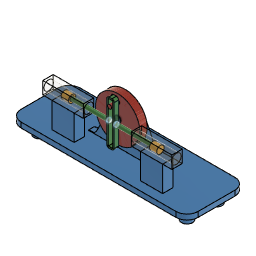
Scotch Yoke Mechanism (Autodesk Fusion 360 design; units mm, degrees)
Autodesk Fusion 360 part; units mm, degrees
note: some values were not read from the file. Set by a fixed rule: which face or edge a step refers to.
sketch "legs" plane through (0, 0, 0) normal (0, 0, 1) x (1, 0, 0) in component "Holder"
  circle A0 centre (-100, -20) radius 7.5
  circle A1 centre (100, -20) radius 7.5
  circle A2 centre (-100, 20) radius 7.5
  circle A3 centre (100, 20) radius 7.5
  dimension "d3" = 15
  dimension "d4" = 15
  dimension "d5" = 15
  dimension "d6" = 15
  measures "d3" diameter of A0
  measures "d4" diameter of A1
  measures "d5" diameter of A2
  measures "d6" diameter of A3
extrude "Extrude1" add sketch "legs" along normal blind 15 makes body 1 at (107.4627, 19.2532, 10) makes body 2 at (-92.5373, 19.2532, 10) makes body 3 at (107.4627, -20.7468, 10) makes body 4 at (-92.5373, -20.7468, 10) in component "Holder"
sketch "plank" plane through (0, 0, 15) normal (0, 0, 1) x (-1, 0, 0) in component "Holder"
  line L0 (120, 40) -> (-120, 40)
  line L1 (-120, 40) -> (-120, -40)
  line L2 (-120, -40) -> (120, -40)
  line L3 (120, -40) -> (120, 40)
  constraint horizontal L0
  constraint vertical L1
  constraint horizontal L2
  constraint vertical L3
extrude "Extrude2" add sketch "plank" along normal blind 7 bodies 1 2 3 4 in component "Holder"
fillet "Fillet1" radius 15 4 edges at (-120, -40, 18.5) (-120, 40, 18.5) (120, 40, 18.5) (120, -40, 18.5) on bodies 1 in component "Holder"
sketch "crank base" plane through (0, 0, 0) normal (0, 1, 0) x (1, 0, 0) in component "Holder"
  spline S0 degree 5 poles (-50, -22) (-49.5881, -22.201) (-48.7779, -22.5509) (-47.6039, -22.9192) (-46.1206, -23.0999) (-44.378, -22.949) (-42.6597, -22.9112) (-40.8151, -23.8091) (-38.6826, -26.4236) (-36.1403, -31.1271) (-33.1188, -37.8246) (-29.5891, -46.0954) (-25.5591, -55.2688) (-21.0666, -64.5249) (-16.1749, -72.9822) (-10.9666, -79.791) (-5.5393, -84.224) (0, -85.7692) (5.5393, -84.224) (10.9666, -79.791) (16.1749, -72.9822) (21.0666, -64.5249) (25.5591, -55.2688) (29.5891, -46.0953) (33.1188, -37.8246) (36.1403, -31.1271) (38.6826, -26.4236) (40.8151, -23.8091) (42.6597, -22.9112) (44.378, -22.949) (46.1206, -23.0999) (47.6039, -22.9192) (48.7779, -22.5509) (49.5881, -22.201) (50, -22) knots 0 0 0 0 0 0 0.033333 0.066667 0.1 0.133333 0.166667 0.2 0.233333 0.266667 0.3 0.333333 0.366667 0.4 0.433333 0.466667 0.5 0.533333 0.566667 0.6 0.633333 0.666667 0.7 0.733333 0.766667 0.8 0.833333 0.866667 0.9 0.933333 0.966667 1 1 1 1 1 1
  line L0 (-50, -22) -> (50, -22)
  point P0 (-45, -23)
  point P1 (-40, -25)
  point P2 (0, -85)
  point P3 (40, -25)
  point P4 (45, -23)
  constraint horizontal L0
sketch "base of crank base" plane through (0, 0, 22) normal (0, 0, 1) x (-1, 0, 0) in component "Holder"
  arc A0 (-105, 40) -> (-120, 25) centre (-105, 25) ccw
  line L0 (-120, 25) -> (-120, -25)
  arc A1 (-120, -25) -> (-105, -40) centre (-105, -25) ccw
  line L1 (-105, -40) -> (105, -40)
  arc A2 (105, -40) -> (120, -25) centre (105, -25) ccw
  line L2 (120, -25) -> (120, 25)
  arc A3 (120, 25) -> (105, 40) centre (105, 25) ccw
  line L3 (105, 40) -> (-105, 40)
  line L4 (50, -4) -> (-50.6051, -4)
  line L5 (-50.6051, -4) -> (-50.6051, 4)
  line L6 (-50.6051, 4) -> (50, 4)
  line L7 (50, 4) -> (50, -4)
  dimension "d16" = 8
  constraint horizontal L4
  constraint vertical L5
  constraint horizontal L6
  constraint vertical L7
  measures "d16" distance of L4.start L6.end
extrude "Extrude4" add sketch "crank base" along normal mid plane 8 bodies 1 in component "Holder"
sketch "Crank" plane through (0, -4, 0) normal (0, -1, 0) x (1, 0, 0) in component "Crank (1)"
  spline S0 degree 5 poles (50, 22) (49.5881, 22.201) (48.7779, 22.5509) (47.6039, 22.9192) (46.1206, 23.0999) (44.378, 22.949) (42.6597, 22.9112) (40.8151, 23.8091) (38.6826, 26.4236) (36.1403, 31.1271) (33.1188, 37.8246) (29.5891, 46.0953) (25.5591, 55.2688) (21.0666, 64.5249) (16.1749, 72.9822) (10.9666, 79.791) (5.5393, 84.224) (0, 85.7692) (-5.5393, 84.224) (-10.9666, 79.791) (-16.1749, 72.9822) (-21.0666, 64.5249) (-25.5591, 55.2688) (-29.5891, 46.0954) (-33.1188, 37.8246) (-36.1403, 31.1271) (-38.6826, 26.4236) (-40.8151, 23.8091) (-42.6597, 22.9112) (-44.378, 22.949) (-46.1206, 23.0999) (-47.6039, 22.9192) (-48.7779, 22.5509) (-49.5881, 22.201) (-50, 22) knots -1 -1 -1 -1 -1 -1 -0.966667 -0.933333 -0.9 -0.866667 -0.833333 -0.8 -0.766667 -0.733333 -0.7 -0.666667 -0.633333 -0.6 -0.566667 -0.533333 -0.5 -0.466667 -0.433333 -0.4 -0.366667 -0.333333 -0.3 -0.266667 -0.233333 -0.2 -0.166667 -0.133333 -0.1 -0.066667 -0.033333 0 0 0 0 0 0
  line L0 (-50, 22) -> (50, 22)
  circle A0 centre (0, 64.9652) radius 30
  dimension "d19" = 60
  measures "d19" diameter of A0
extrude "Extrude1'" add sketch "Crank" along normal blind 10 separate body contours S0 A0 | S0 A0 makes body 5 in component "Crank (1)"
sketch "Holder pin" plane through (0, -14, 0) normal (0, -1, 0) x (1, 0, 0) in component "Crank (1)"
  circle A0 centre (0, 64.9652) radius 30
  circle A1 centre (0, 64.9652) radius 4
  dimension "d22" = 8
  constraint concentric A0 A1
  measures "d22" diameter of A1
extrude "Extrude2'" cut sketch "Holder pin" against normal blind 103 contours A1 bodies 5 in component "Crank (1)"
extrude "Extrude5" add sketch "Holder pin" along normal blind -10 and the other way blind -3 contours A1 bodies 1 in component "Holder"
move_face "OffsetFaces1" offset -0.3 1 faces at (3.9801, -8.3333, 64.567) on bodies 1 in component "Holder"
sketch "Connecting Rod" plane through (0, -14, 0) normal (0, -1, 0) x (1, 0, 0) in component "Slider"
  line L0 (-5, 95) -> (5, 95)
  line L1 (5, 95) -> (5, 35)
  line L2 (5, 35) -> (-5, 35)
  line L3 (-5, 35) -> (-5, 95)
  line L4 (-3, 37) -> (-3, 93)
  line L5 (-3, 93) -> (3, 93)
  line L6 (3, 93) -> (3, 37)
  line L7 (3, 37) -> (-3, 37)
  dimension "d33" = 2
  constraint horizontal L0
  constraint vertical L1
  constraint horizontal L2
  constraint vertical L3
extrude "Extrude4'" add sketch "Connecting Rod" along normal blind 10 and the other way blind -4 separate body makes body 6 in component "Slider"
fillet "Fillet2" radius 3 4 edges at (5, -21, 95) (-5, -21, 95) (-5, -21, 35) (5, -21, 35) on bodies 6 in component "Slider"
sketch "Right bar" plane through (5, 0, 0) normal (1, 0, 0) x (0, 1, 0) in component "Slider"
  line L0 (-24, 38) -> (-18, 38)
  line L1 (-18, 38) -> (-18, 92)
  line L2 (-18, 92) -> (-24, 92)
  line L3 (-24, 92) -> (-24, 38)
  circle A0 centre (-21, 65) radius 3
  dimension "d53" = 6
  measures "d53" diameter of A0
sketch "Left Bar" plane through (-5, 0, 0) normal (-1, 0, 0) x (0, -1, 0) in component "Slider"
  line L0 (18, 38) -> (24, 38)
  line L1 (24, 38) -> (24, 92)
  line L2 (24, 92) -> (18, 92)
  line L3 (18, 92) -> (18, 38)
  circle A0 centre (21, 65) radius 3
  dimension "d54" = 6
  measures "d54" diameter of A0
sketch "Connecting pin" plane through (0, -14, 0) normal (0, -1, 0) x (1, 0, 0) in component "Crank (1)"
  circle A0 centre (0, 85) radius 2.75
  dimension "d67" = 5.5
  measures "d67" diameter of A0
extrude "Extrude5'" add sketch "Connecting pin" along normal blind 11 bodies 5 in component "Crank (1)"
sketch "left piston" plane through (0, 0, 0) normal (0, 1, 0) x (1, 0, 0) in component "Left piston"
  line L0 (-55, -70) -> (-65, -70)
  line L1 (-65, -70) -> (-65, -60)
  line L2 (-65, -60) -> (-55, -60)
  line L3 (-55, -60) -> (-55, -70)
  line L4 (0, -110) -> (0, -15) construction
  constraint horizontal L0
  constraint vertical L1
  constraint horizontal L2
  constraint vertical L3
  constraint vertical L4
extrude "Extrude1''" add sketch "left piston" along normal blind -16 and the other way blind 26 separate body makes body 7 in component "Left piston"
fillet "Fillet1'" radius 5 4 edges at (-60, -26, 70) (-60, -16, 70) (-60, -16, 60) (-60, -26, 60) on bodies 7 in component "Left piston"
extrude "Extrude2''" cut sketch "Left Bar" along normal blind 55 contours A0 bodies 7 in component "Left piston"
extrude "Extrude7" add sketch "Left Bar" along normal blind 55 contours A0 bodies 6 in component "Slider"
sketch "right piston" plane through (0, 0, 0) normal (0, 1, 0) x (1, 0, 0) in component "Right piston"
  line L0 (55, -70) -> (65, -70)
  line L1 (65, -70) -> (65, -60)
  line L2 (65, -60) -> (55, -60)
  line L3 (55, -60) -> (55, -70)
  constraint horizontal L0
  constraint vertical L1
  constraint horizontal L2
  constraint vertical L3
extrude "Extrude1'''" add sketch "right piston" along normal blind -16 and the other way blind 26 separate body makes body 8 in component "Right piston"
extrude "Extrude2'''" cut sketch "Right bar" along normal blind 55 contours A0 bodies 8 in component "Right piston"
extrude "Extrude8" add sketch "Right bar" along normal blind 55 contours A0 bodies 6 in component "Slider"
fillet "Fillet1''" radius 5 4 edges at (60, -26, 70) (60, -16, 70) (60, -16, 60) (60, -26, 60) on bodies 8 in component "Right piston"
move_face "OffsetFaces1'" offset -0.3 1 faces at (-23.3333, -18.0037, 64.8505) on bodies 6 in component "Slider"
move_face "OffsetFaces2" offset -0.3 1 faces at (41.6667, -23.9963, 65.1495) on bodies 6 in component "Slider"
sketch "left bar holder" plane through (0, 0, 0) normal (0, 1, 0) x (1, 0, 0) in component "Left bar holder"
  line L0 (-87.5, -58.5) -> (-38.5, -58.5)
  line L1 (-38.5, -71.5) -> (-87.5, -71.5)
  line L2 (-32.5, -71.5) -> (-32.5, -58.5)
  line L3 (-32.5, -58.5) -> (-87.5, -58.5)
  line L4 (-87.5, -58.5) -> (-87.5, -71.5)
  line L5 (-87.5, -71.5) -> (-32.5, -71.5)
extrude "Extrude8'" add sketch "left bar holder" along normal blind -16 and the other way blind 26 separate body makes body 9 in component "Left bar holder"
sketch "right bar holder" plane through (0, 0, 0) normal (0, 1, 0) x (1, 0, 0) in component "Right bar holder"
  line L0 (87.5, -58.5) -> (32.5, -58.5)
  line L1 (32.5, -58.5) -> (32.5, -71.5)
  line L2 (32.5, -71.5) -> (87.5, -71.5)
  line L3 (87.5, -71.5) -> (87.5, -58.5)
extrude "Extrude1''''" add sketch "right bar holder" along normal blind -16 and the other way blind 26 separate body makes body 10 in component "Right bar holder"
extrude "Extrude10" add 2 faces at (-36.5, -22.6667, 71.5) (-54.8333, -19.3333, 71.5) along direction (0, 0, 1) blind 2 on bodies 9 bodies 9 in component "Left bar holder"
extrude "Extrude11" add 1 faces at (-50.8333, -26, 68.5) along direction (0, -1, 0) blind 2 on bodies 9 bodies 9 in component "Left bar holder"
extrude "Extrude12" add 1 faces at (-69.1667, -24, 58.5) along direction (0, 0, -1) blind 2 on bodies 9 bodies 9 in component "Left bar holder"
extrude "Extrude13" add 1 faces at (-50.8333, -16, 62.1667) along direction (0, 1, 0) blind 2 on bodies 9 bodies 9 in component "Left bar holder"
hole "Hole5" at (-32.5, -21, 65) direction (-1, 0, 0) diameter 13 depth 54 tip angle 180 bodies 9 in component "Left bar holder"
extrude "Extrude3" add 1 faces at (50.8333, -22.6667, 71.5) along direction (0, 0, 1) blind 2 on bodies 10 bodies 10 in component "Right bar holder"
extrude "Extrude4''" add 1 faces at (50.8333, -26, 63.5) along direction (0, -1, 0) blind 2 on bodies 10 bodies 10 in component "Right bar holder"
extrude "Extrude5''" add 1 faces at (69.1667, -24, 58.5) along direction (0, 0, -1) blind 2 on bodies 10 bodies 10 in component "Right bar holder"
extrude "Extrude6" add 1 faces at (50.8333, -16, 62.1667) along direction (0, 1, 0) blind 2 on bodies 10 bodies 10 in component "Right bar holder"
hole "Hole2" at (32.5, -21, 65) direction (1, 0, 0) diameter 13 depth 54 tip angle 180 bodies 10 in component "Right bar holder"
sketch "mini holders" plane through (0, 0, 22) normal (0, 0, 1) x (-1, 0, 0) in component "Holder"
  line L0 (-50, 4) -> (50, 4)
  line L1 (50, 4) -> (50, -4)
  line L2 (50, -4) -> (-50, -4)
  line L3 (-50, -4) -> (-50, 4)
  arc A0 (-105, 40) -> (-120, 25) centre (-105, 25) ccw
  line L4 (-120, 25) -> (-120, -25)
  arc A1 (-120, -25) -> (-105, -40) centre (-105, -25) ccw
  line L5 (-105, -40) -> (105, -40)
  arc A2 (105, -40) -> (120, -25) centre (105, -25) ccw
  line L6 (120, -25) -> (120, 25)
  arc A3 (120, 25) -> (105, 40) centre (105, 25) ccw
  line L7 (105, 40) -> (-105, 40)
  line L8 (-45, 14) -> (-75, 14)
  line L9 (-75, 14) -> (-75, 28)
  line L10 (-75, 28) -> (-45, 28)
  line L11 (-45, 28) -> (-45, 14)
  line L12 (75, 14) -> (45, 14)
  line L13 (45, 14) -> (45, 28)
  line L14 (45, 28) -> (75, 28)
  line L15 (75, 28) -> (75, 14)
  constraint horizontal L8
  constraint vertical L9
  constraint horizontal L10
  constraint vertical L11
  constraint horizontal L12
  constraint vertical L13
  constraint horizontal L14
  constraint vertical L15
extrude "Extrude6'" add sketch "mini holders" along normal blind 34.5 contours L8 L9 L10 L11 | L12 L13 L14 L15 bodies 1 in component "Holder"
component "Holder" placed x (1, 0, 0) y (0, 1, 0) z (0, 0, 1) at (0, 0, 0)
component "Crank (1)" placed x (1, 0, 0) y (0, 1, 0) z (0, 0, 1) at (0, 0, 0)
component "Slider" placed x (1, 0, 0) y (0, 1, 0) z (0, 0, 1) at (0.25, 0, 0)
component "Left piston" placed x (1, 0, 0) y (0, 1, 0) z (0, 0, 1) at (0.25, 0, 0)
component "Right piston" placed x (1, 0, 0) y (0, 1, 0) z (0, 0, 1) at (0, 0, 0)
component "Left bar holder" placed x (1, 0, 0) y (0, 1, 0) z (0, 0, 1) at (0, 0, 0)
component "Right bar holder" placed x (1, 0, 0) y (0, 1, 0) z (0, 0, 1) at (0, 0, 0)
named bodies: "Holder", "Left leg behind", "Right leg front", "Left leg front", "Crank", "Slider", "Right piston", "Left bar holder", "Right bar holder"
